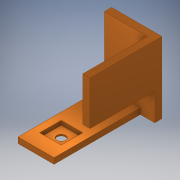
# Autodesk Inventor part: Slider
Saved by Autodesk Inventor 2017 (Build 210142000, 142)
## iProperties
Created: 2017-05-30
Part Number: Slider
Material: Gold
Document SubType Name: Modeling
Designer: sensor
Density: 19.3 g/cm^3
Appearance: Metal 1600F Hot
Author: sensor
Autodesk Inventor part; units mm, degrees
ref_plane "YZ Plane" through (0, 0, 0) normal (1, 0, 0) x (0, 1, 0)
ref_plane "XZ Plane" through (0, 0, 0) normal (0, 1, 0) x (-1, 0, 0)
ref_plane "XY Plane" through (0, 0, 0) normal (0, 0, 1) x (1, 0, 0)
sketch "Sketch1" plane through (0, 0, 0) normal (0, 1, 0) x (-1, 0, 0)
  line L0 (0, 0) -> (25, 0)
  line L1 (25, 0) -> (25, 65)
  line L2 (25, 65) -> (0, 65)
  line L3 (0, 65) -> (0, 0)
  circle A0 centre (12.5, 47.5) radius 3
  circle A1 centre (12.5, 17.5) radius 3
  dimension "d8" = 25
  dimension "d9" = 65
  dimension "d10" = 6
  dimension "d11" = 6
  dimension "d12" = 12.5
  dimension "d13" = 12.5
  dimension "d14" = 17.5
  dimension "d15" = 17.5
  constraints: 8 end point, 2 centre point, 2 parallel, 1 horizontal, 1 perpendicular
  measures "d8" distance of L1.end L2.end
  measures "d9" distance of L0.end L1.end
  measures "d10" diameter of A0
  measures "d11" diameter of A1
  measures "d12" distance from line of L3 A0.centre
  measures "d13" distance from line of A1.centre L3
  measures "d14" distance from line of A0.centre L2
  measures "d15" distance from line of L0 A1.centre
extrude "Extrusion1" add sketch "Sketch1" along normal blind 4
sketch "Sketch2" plane through (0, 4, 0) normal (0, 1, 0) x (1, 0, 0)
  line L0 (0, -65) -> (0, 0) projected
  line L1 (0, 0) -> (-25, 0) projected
  line L2 (0, -5) -> (-25, -5)
  line L3 (-25, -5) -> (-25, 0)
  line L4 (-25, 0) -> (0, 0)
  line L5 (0, 0) -> (0, -5)
  dimension "d18" = 5
  constraints: 8 end point, 2 parallel, 1 horizontal, 1 perpendicular, 1 point on line
  measures "d18" distance of L0.end L2.start
extrude "Extrusion2" add sketch "Sketch2" along normal blind 15
sketch "Sketch3" plane through (-25, 4, 5) normal (0, 0, 1) x (1, 0, 0)
  circle A0 centre (17.5, 7.5) radius 2.5
  circle A1 centre (7.5, 7.5) radius 2.5
  line L0 (25, 0) -> (25, 15) projected
  line L1 (0, 0) -> (0, 15) projected
  line L2 (0, 0) -> (25, 0) projected
  point P0 (25, -4)
  dimension "d21" = 5
  dimension "d22" = 5
  dimension "d23" = 7.5
  dimension "d24" = 7.5
  dimension "d25" = 7.5
  dimension "d26" = 7.5
  dimension "d27" = 10
  constraints: 2 centre point
  measures "d21" diameter of A0
  measures "d22" diameter of A1
  measures "d23" distance from line of L0 A0.centre
  measures "d24" distance from line of L1 A1.centre
  measures "d25" distance from line of L2 A0.centre
  measures "d26" distance from line of L2 A1.centre
  measures "d27" distance of A1.centre A0.centre
hole "Hole1" at (-7.5, 11.5, 5) at (-17.5, 11.5, 5) direction (0, 0, -1) diameter 5.86 end through all
sketch "Sketch4" plane through (0, 4, 0) normal (0, 1, 0) x (1, 0, 0)
  line L0 (-20, -55) -> (-5, -55)
  line L1 (-5, -55) -> (-5, -40)
  line L2 (-5, -40) -> (-20, -40)
  line L3 (-20, -40) -> (-20, -55)
  line L4 (-25, -65) -> (0, -65) projected
  line L5 (0, -65) -> (0, -5) projected
  point P0 (0, 0)
  dimension "d35" = 10
  dimension "d36" = 15
  dimension "d37" = 15
  dimension "d38" = 5
  constraints: 8 end point, 2 parallel, 1 horizontal, 1 perpendicular
  measures "d35" distance between parallel lines of L4 L0
  measures "d36" distance of L1.end L2.end
  measures "d37" distance of L2.end L0.start
  measures "d38" distance between parallel lines of L5 L1
extrude "Extrusion3" cut sketch "Sketch4" against normal blind 3
sketch "Sketch6" plane through (0, 4, 0) normal (0, 1, 0) x (1, 0, 0)
  line L0 (-20, -25) -> (-5, -25)
  line L1 (-5, -25) -> (-5, -10)
  line L2 (-5, -10) -> (-20, -10)
  line L3 (-20, -10) -> (-20, -25)
  line L4 (0, -65) -> (0, -5) projected
  line L5 (-20, -40) -> (-5, -40) projected
  point P0 (0, 0)
  point P1 (-20, -40)
  dimension "d41" = 15
  dimension "d42" = 15
  dimension "d43" = 5
  dimension "d44" = 30
  constraints: 8 end point, 2 parallel, 1 horizontal, 1 perpendicular
  measures "d41" distance of L2.end L0.start
  measures "d42" distance of L0.start L0.end
  measures "d43" distance between parallel lines of L4 L1
  measures "d44" distance between parallel lines of L2 L5
extrude "Extrusion4" cut sketch "Sketch6" against normal blind 3
sketch "Sketch9" plane through (0, 19, 0) normal (0, 1, 0) x (1, 0, 0)
  line L0 (0, 0) -> (-25, 0) projected
  line L1 (-25, 0) -> (-25, -5) projected
  line L2 (0, 0) -> (-25, 0)
  line L3 (-25, 0) -> (-25, -5)
  line L4 (-25, -5) -> (0, -5)
  line L5 (0, -5) -> (0, 0)
  constraints: 8 end point, 2 parallel, 1 horizontal, 1 perpendicular
extrude "Extrusion7" add sketch "Sketch9" along normal blind 23
sketch "Sketch12" plane through (0, 0, 65) normal (1, 0, 0) x (0, 0, -1)
  line L0 (60, 42) -> (65, 42) projected
  line L1 (65, 0) -> (60, 0)
  line L2 (60, 0) -> (60, 42)
  line L3 (60, 42) -> (65, 42)
  line L4 (65, 42) -> (65, 0)
  constraints: 8 end point, 2 parallel, 1 horizontal, 1 perpendicular
extrude "Extrusion8" add sketch "Sketch12" along normal blind 10
sketch "Sketch13" plane through (-25, 4, 5) normal (0, 0, 1) x (1, 0, 0)
  line L0 (35, -4) -> (35, 38) projected
  line L1 (0, 38) -> (35, 38) projected
  line L2 (35, 15) -> (30, 15)
  line L3 (30, 15) -> (30, 38)
  line L4 (30, 38) -> (35, 38)
  line L5 (35, 38) -> (35, 15)
  point P0 (25, -4)
  dimension "d56" = 5
  dimension "d57" = 23
  constraints: 8 end point, 2 parallel, 2 point on line, 1 horizontal, 1 perpendicular
  measures "d56" distance of L2.start L2.end
  measures "d57" distance of L2.end L3.end
extrude "Extrusion9" add sketch "Sketch13" along normal blind 45
sketch "Sketch14" plane through (0, 42, 0) normal (0, 1, 0) x (1, 0, 0)
  line L0 (10, 0) -> (10, -50) projected
  line L1 (5, -50) -> (10, -50) projected
  line L2 (10, -50) -> (5, -50)
  line L3 (-25, -5) -> (5, -5) projected
  line L4 (5, -50) -> (5, -5)
  line L5 (5, -5) -> (-25, -5)
  line L6 (-25, 0) -> (10, 0) projected
  line L7 (-25, -5) -> (-25, 0)
  line L8 (-25, 0) -> (10, 0)
  line L9 (10, 0) -> (10, -50)
  point P0 (0, 0)
  constraints: 12 end point, 3 collinear, 3 perpendicular
extrude "Extrusion10" add sketch "Sketch14" along normal blind 7.5
body "Solid1"
